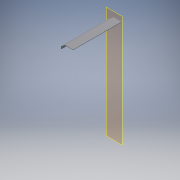
# Autodesk Inventor part: Drive BaseFront
Saved by Autodesk Inventor 2017 (Build 210142000, 142)
## iProperties
Created: 2017-04-25
Part Number: Drive BaseFront
Material: Generic
Document SubType Name: Modeling
Designer: admin
Density: 1 g/cm^3
Appearance: Default
Author: admin
Autodesk Inventor part; units mm, degrees
ref_plane "YZ Plane" through (0, 0, 0) normal (1, 0, 0) x (0, 1, 0)
ref_plane "XZ Plane" through (0, 0, 0) normal (0, 1, 0) x (-1, 0, 0)
ref_plane "XY Plane" through (0, 0, 0) normal (0, 0, 1) x (1, 0, 0)
ref_plane "Work Plane1" through (0, 0, 0) normal (0, 0, 1) x (1, 0, 0)
sketch "Sketch1" plane through (0, 0, 0) normal (0, 0, 1) x (1, 0, 0)
  line L0 (41.7899, 406.4) -> (106.8774, 406.4) projected
  line L1 (14.8024, 385.8381) -> (41.7899, 406.4) projected
  line L2 (106.8774, 403.225) -> (42.8616, 403.225)
  line L3 (42.8616, 403.225) -> (16.7266, 383.3126)
  line L4 (106.8774, 406.4) -> (106.8774, 403.225)
  line L5 (11.6274, 361.95) -> (11.6274, 80.1687) projected
  line L6 (16.7266, 383.3126) -> (11.6274, 379.4275)
  line L7 (14.8024, 385.8381) -> (8.4524, 381)
  line L8 (11.6274, 361.95) -> (11.6274, 379.4275)
  line L9 (11.6274, 361.95) -> (11.6274, 80.1687) projected
  line L10 (8.4524, 361.95) -> (8.4524, 80.1687) projected
  line L11 (11.6274, 361.95) -> (8.4524, 361.95) projected
  line L12 (8.4524, 361.95) -> (8.4524, 381)
  point P0 (0, 0)
  dimension "d0" = 3.175
  constraints: 14 end point, 3 vertical, 1 collinear, 1 other
  measures "d0" distance between parallel lines of L0 L2
extrude "Extrusion1" add sketch "Sketch1" along normal blind 387.35
body "Solid1"
